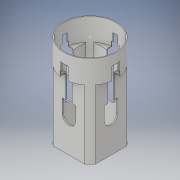
# Autodesk Inventor part: Hull2
Saved by Autodesk Inventor 2018.2 (Build 222227000, 227)
## iProperties
Created: 2017-12-27
Part Number: Hull2
Material: Generic
Document SubType Name: Modeling
Designer: Suchanek
Density: 1 g/cm^3
Appearance: Default
Mass: 15.1041 g
Surface Area: 312.787 cm^2
Volume: 15.1041 cm^3
Author: Suchanek
Autodesk Inventor part; units mm, degrees
ref_plane "YZ Plane" through (0, 0, 0) normal (1, 0, 0) x (0, 1, 0)
ref_plane "XZ Plane" through (0, 0, 0) normal (0, 1, 0) x (-1, 0, 0)
ref_plane "XY Plane" through (0, 0, 0) normal (0, 0, 1) x (1, 0, 0)
sketch "Sketch1" plane through (0, 0, 0) normal (0, 0, 1) x (1, 0, 0)
  line L0 (0, 0) -> (33, 0)
  line L1 (33, 0) -> (33, 1)
  line L2 (33, 1) -> (0, 1)
  line L3 (0, 1) -> (0, 0)
  line L4 (33, 0) -> (32, 0)
  line L5 (32, 0) -> (32, 115)
  line L6 (32, 115) -> (33, 115)
  line L7 (33, 115) -> (33, 0)
  line L8 (33, 115) -> (0, 115)
  line L9 (0, 115) -> (0, 115)
  line L10 (0, 115) -> (33, 115)
  line L11 (33, 115) -> (33, 115)
  line L12 (0, 115) -> (0, 1)
  line L13 (-5, 105) -> (5, 105)
  line L14 (5, 105) -> (5, 5)
  line L15 (5, 5) -> (-5, 5)
  line L16 (-5, 5) -> (-5, 105)
  dimension "d0" = 33
  dimension "d1" = 1
  dimension "d2" = 1
  dimension "d3" = 115
  dimension "d4" = 33
  dimension "d5" = 0
  dimension "d6" = 10
  dimension "d7" = 100
  dimension "d8" = 4
  constraints: 34 end point, 8 equal length, 4 perpendicular, 3 horizontal, 1 other
  measures "d0" distance of L2.end L1.end
  measures "d1" distance of L1.end L0.end
  measures "d2" distance of L5.end L6.end
  measures "d3" distance of L4.end L5.end
  measures "d4" distance of L10.end L9.end
  measures "d5" distance of L9.end L8.end
  measures "d6" distance of L14.end L15.end
  measures "d7" distance of L15.end L13.start
  measures "d8" distance from line of L1.end L15
sketch "Sketch2" plane through (0, 0, 0) normal (1, 0, 0) x (0, 1, 0)
  line L0 (102.5, 5) -> (5, 5)
  line L1 (5, 5) -> (5, -5)
  line L2 (5, -5) -> (102.5, -5)
  line L3 (102.5, -5) -> (102.5, 5)
  line L4 (0, 0) -> (0, -10)
  line L5 (0, 0) -> (115, 0)
  dimension "d9" = 10
  dimension "d10" = 5
  dimension "d12" = 115
  dimension "d13" = 10
  dimension "d14" = 97.5
  constraints: 12 end point, 2 horizontal, 2 parallel, 1 perpendicular, 1 vertical, 1 other
  measures "d9" distance of L4.start L4.end
  measures "d10" distance between parallel lines of L1 L4
  measures "d12" distance of L4.start L5.end
  measures "d13" distance between parallel lines of L0 L2
  measures "d14" distance of L1.end L2.end
extrude "Extrusion1" add sketch "Sketch2" along normal mid plane 10
revolve "Revolution1" add sketch "Sketch1" angle 360 about axis through (0, 115, 0) along (0, -1, 0) contours L3 L2 L5 L0 | L5 L2 L1 L0 | L5 L6 L7 L2
sketch "Sketch3" plane through (-5, 5, 5) normal (0, 0, 1) x (1, 0, 0)
  line L0 (0, 97.5) -> (10, 97.5) projected
  line L1 (10, 97.5) -> (10, 0) projected
  line L2 (0, 97.5) -> (10, 97.5)
  line L3 (10, 97.5) -> (10, 0)
  line L4 (10, 0) -> (0, 0)
  line L5 (0, 0) -> (0, 97.5)
  point P0 (5, -5)
  dimension "d18" = 97.5
  constraints: 8 end point, 2 parallel, 1 horizontal, 1 perpendicular
  measures "d18" distance of L2.end L1.end
extrude "Extrusion2" cut sketch "Sketch3" along normal mid plane 200
sketch "Sketch4" plane through (5, 0, 0) normal (1, 0, 0) x (0, 0, -1)
  line L0 (-5, 102.5) -> (-5, 5) projected
  line L1 (-5, 102.5) -> (5, 102.5)
  line L2 (5, 102.5) -> (5, 5)
  line L3 (5, 5) -> (-5, 5)
  line L4 (-5, 5) -> (-5, 102.5)
  point P0 (0, 0)
  dimension "d21" = 10
  dimension "d70" = 97.5
  constraints: 8 end point, 2 parallel, 1 horizontal, 1 perpendicular, 1 point on line
  measures "d21" distance of L2.end L3.end
  measures "d70" distance between parallel lines of L3 L1
extrude "Extrusion3" cut sketch "Sketch4" along normal mid plane 200
sketch "Sketch5" plane through (-32.619013, 5, -5) normal (0, 0, 1) x (1, 0, 0)
  line L0 (65.238026, 97.5) -> (64.225974, 97.5)
  line L1 (65.238026, 97.5) -> (55.238026, 97.5)
  line L2 (55.238026, 97.5) -> (55.238026, 87.5)
  line L3 (55.238026, 87.5) -> (65.238026, 87.5)
  line L4 (65.238026, 87.5) -> (65.238026, 97.5)
  line L5 (0, 97.5) -> (-0.380987, 97.5)
  line L6 (0, 97.5) -> (10, 97.5)
  line L7 (10, 97.5) -> (10, 87.5)
  line L8 (10, 87.5) -> (0, 87.5)
  line L9 (0, 87.5) -> (0, 97.5)
  circle A0 centre (7.5, 90) radius 1
  circle A1 centre (57.738026, 90) radius 1
  point P0 (32.619013, -5)
  dimension "d26" = 10
  dimension "d27" = 10
  dimension "d56" = 10
  dimension "d57" = 10
  dimension "d58" = 2
  dimension "d59" = 2.5
  dimension "d60" = 2.5
  dimension "d61" = 2
  dimension "d62" = 2.5
  dimension "d63" = 2.5
  constraints: 16 end point, 4 parallel, 2 centre point, 2 horizontal, 2 perpendicular
  measures "d26" distance of L3.end L2.end
  measures "d27" distance of L2.end L1.end
  measures "d56" distance of L7.end L8.end
  measures "d57" distance of L6.end L7.end
  measures "d58" diameter of A0
  measures "d59" distance from line of L7 A0.centre
  measures "d60" distance from line of L8 A0.centre
  measures "d61" diameter of A1
  measures "d62" distance from line of A1.centre L2
  measures "d63" distance from line of A1.centre L3
extrude "Extrusion4" add sketch "Sketch5" along normal blind 2
sketch "Sketch7" plane through (0, 1, 0) normal (0, 1, 0) x (1, 0, 0)
  line L0 (0, 0) -> (-26.5, 0)
  line L1 (-26.5, 0) -> (-26.5, 26.5)
  line L2 (-26.5, 26.5) -> (0, 26.5)
  line L3 (0, 26.5) -> (0, 0)
  line L4 (-26.5, 26.5) -> (26.5, 26.5)
  line L5 (26.5, 26.5) -> (26.5, 33.5)
  line L6 (26.5, 33.5) -> (-26.5, 33.5)
  line L7 (-26.5, 33.5) -> (-26.5, 26.5)
  line L8 (26.5, 26.5) -> (33.5, 26.5)
  line L9 (33.5, 26.5) -> (33.5, -26.5)
  line L10 (33.5, -26.5) -> (26.5, -26.5)
  line L11 (26.5, -26.5) -> (26.5, 26.5)
  line L12 (-26.5, 26.5) -> (-33.5, 26.5)
  line L13 (-33.5, 26.5) -> (-33.5, -26.5)
  line L14 (-33.5, -26.5) -> (-26.5, -26.5)
  line L15 (-26.5, -26.5) -> (-26.5, 26.5)
  line L16 (-26.5, -26.5) -> (26.5, -26.5)
  line L17 (26.5, -26.5) -> (26.5, -33.5)
  line L18 (26.5, -33.5) -> (-26.5, -33.5)
  line L19 (-26.5, -33.5) -> (-26.5, -26.5)
  dimension "d36" = 26.5
  dimension "d37" = 26.5
  dimension "d38" = 53
  dimension "d39" = 7
  dimension "d40" = 7
  dimension "d41" = 53
  dimension "d42" = 7
  dimension "d43" = 53
  dimension "d44" = 53
  dimension "d45" = 7
  constraints: 40 end point, 10 parallel, 5 horizontal, 5 perpendicular
  measures "d36" distance of L1.end L2.end
  measures "d37" distance of L0.end L1.end
  measures "d38" distance of L6.end L5.end
  measures "d39" distance of L5.end L4.end
  measures "d40" distance of L9.end L10.end
  measures "d41" distance of L8.end L9.end
  measures "d42" distance of L14.end L13.end
  measures "d43" distance of L13.end L12.end
  measures "d44" distance of L17.end L18.end
  measures "d45" distance of L16.end L17.end
extrude "Extrusion6" cut sketch "Sketch7" along normal blind 85 and the other way blind 5 contours L15 L14 L13 L12 L1 | L2 L7 L6 L5 L4 | L16 L17 L18 L19 | L8 L9 L10 L11
sketch "Sketch8" plane through (-17.937391, 1, 26.5) normal (0, 1, 0) x (1, 0, 0)
  point P0 (17.937391, 26.5)
sketch "Sketch9" plane through (-17.937391, 1, 26.5) normal (0, 1, 0) x (1, 0, 0)
  line L0 (1.437391, 43) -> (34.437391, 43)
  line L1 (34.437391, 43) -> (34.437391, 10)
  line L2 (34.437391, 10) -> (1.437391, 10)
  line L3 (1.437391, 10) -> (1.437391, 43)
  line L4 (35.874782, 53) -> (0, 53)
  line L5 (-8.562609, 6.83404) -> (-8.562609, 46.16596)
  line L6 (0, 0) -> (35.874782, 0)
  line L7 (44.437391, 8.562609) -> (44.437391, 44.437391)
  point P0 (17.937391, 26.5)
  dimension "d50" = 10
  dimension "d51" = 10
  dimension "d52" = 10
  dimension "d53" = 10
  constraints: 8 end point, 2 parallel, 1 horizontal, 1 perpendicular
  measures "d50" distance between parallel lines of L4 L0
  measures "d51" distance between parallel lines of L5 L3
  measures "d52" distance between parallel lines of L6 L2
  measures "d53" distance between parallel lines of L7 L1
extrude "Extrusion7" cut sketch "Sketch9" against normal blind 10
pattern_circular "Circular Pattern1" count 4 over 360 about axis through (0, 57.5, 0) along (0, -1, 0) of "Extrusion4"
sketch "Náčrt13" plane through (0, 115, 0) normal (0, 1, 0) x (1, 0, 0)
  point P0 (0, 0)
sketch "Náčrt14" plane through (-19.66596, 0, -26.5) normal (0, -1, 0) x (1, 0, 0)
  line L0 (-6.83404, 8.562609) -> (-6.83404, 44.437391)
  line L1 (-5.33404, 26.5) -> (-5.33404, 47.151249)
  arc A0 (-6.83404, 44.437391) -> (-6.83404, 8.562609) centre (19.66596, 26.5) ccw
  line L2 (-5.33404, 47.151249) -> (-6.83404, 44.437391)
  arc A1 (-11.941001, 21.5) -> (-6.83404, 8.562609) centre (19.66596, 26.5) ccw
  line L3 (-6.83404, 44.437391) -> (-6.83404, 8.562609)
  line L4 (-6.83404, 8.562609) -> (-5.33404, 4.959341)
  circle A2 centre (19.66596, 26.5) radius 33
  line L5 (-5.33404, 4.959341) -> (-5.33404, 26.5)
  point P0 (-11.042345, 35.5)
  point P1 (-11.042345, 17.5)
  dimension "d88" = 25
  constraints: 10 end point, 2 parallel, 1 point on line, 1 vertical, 2 other
  measures "d88" distance of point (19.666, 26.5) L1.start
extrude "Vysunutí9" add sketch "Náčrt14" against normal blind 87 contours L0 L2 L1 L5 L4
sketch "Náčrt15" plane through (0, 86, 0) normal (0, -1, 0) x (1, 0, 0)
  point P0 (0, 0)
sketch "Náčrt16" plane through (0, 86, 0) normal (0, -1, 0) x (1, 0, 0)
  line L0 (-31.606961, 5) -> (-32.619013, 5)
  arc A0 (-26.5, 19.66596) -> (-32.619013, 5) centre (0, 0) ccw
  line L1 (-26.5, 5) -> (-32.619013, 5)
  line L2 (-32.619013, 5) -> (-26.5, 5)
  line L3 (-26.5, 19.66596) -> (-26.5, 17.937391)
  line L4 (-26.5, 19.66596) -> (-32.619013, 5)
  line L5 (-26.5, 5) -> (-26.5, 19.66596)
  point P0 (0, 0)
  constraints: 8 end point, 1 collinear, 1 perpendicular, 1 point on line
extrude "Vysunutí10" add sketch "Náčrt16" against normal blind 1 contours L0 L4 L3 L5 L1
sketch "Náčrt17" plane through (0, 86, 0) normal (0, -1, 0) x (1, 0, 0)
  line L0 (-26.5, -17.937391) -> (-26.5, -19.66596)
  line L1 (-26.5, -5) -> (-26.5, -19.66596)
  line L2 (-26.5, -19.66596) -> (-30.211599, -12.140082)
  line L3 (-30.211599, -12.140082) -> (-31.970794, -5)
  line L4 (-31.970794, -5) -> (-26.5, -5)
  point P0 (0, 0)
  constraints: 8 end point, 1 perpendicular, 1 vertical
extrude "Vysunutí11" add sketch "Náčrt17" against normal blind 1
sketch "Náčrt18" plane through (-19.66596, 0, -26.5) normal (0, -1, 0) x (1, 0, 0)
  line L0 (0, 1.5) -> (41.20662, 1.5)
  circle A0 centre (19.66596, 26.5) radius 33
  line L1 (37.603352, 0) -> (1.728569, 0)
  line L2 (41.20662, 1.5) -> (37.603352, 0)
  line L3 (37.603352, 0) -> (1.728569, 0)
  line L4 (0, 1.5) -> (-1.874699, 1.5)
  line L5 (0, 0) -> (1.728569, 0)
  line L6 (-1.874699, 1.5) -> (1.728569, 0)
  dimension "d95" = 1.5
  constraints: 10 end point, 2 horizontal, 2 point on circle, 1 collinear
  measures "d95" distance of L5.start L0.start
extrude "Vysunutí12" add sketch "Náčrt18" against normal blind 87 contours L0 L2 L1 L6 L4
sketch "Náčrt19" plane through (0, 86, 0) normal (0, -1, 0) x (1, 0, 0)
  line L0 (-19.66596, -26.5) -> (-17.937391, -26.5)
  line L1 (-5, -26.5) -> (-19.66596, -26.5)
  line L2 (-19.66596, -26.5) -> (-9.21923, -31.085485)
  line L3 (-9.21923, -31.085485) -> (-5.463084, -31.92763)
  line L4 (-5.463084, -31.92763) -> (-5, -32.031455)
  line L5 (-5, -32.031455) -> (-5, -26.5)
  line L6 (17.937391, -26.5) -> (19.66596, -26.5)
  line L7 (18.386912, -26.5) -> (11.546452, -30.567242)
  line L8 (11.546452, -30.567242) -> (5, -32.031455)
  line L9 (5, -31.606961) -> (5, -26.5)
  line L10 (5, -32.031455) -> (5, -26.5)
  line L11 (5, -26.5) -> (18.386912, -26.5)
  point P0 (0, 0)
  constraints: 18 end point, 3 point on line, 2 collinear, 1 perpendicular, 1 vertical
extrude "Vysunutí13" add sketch "Náčrt19" against normal blind 1
sketch "Náčrt23" plane through (-19.66596, 0, 26.5) normal (0, -1, 0) x (1, 0, 0)
  line L0 (1.728569, 0) -> (0, 0)
  line L1 (-1.645269, -1.5) -> (1.728569, 0)
  line L2 (-1.645269, -1.5) -> (40.94385, -1.5)
  line L3 (40.94385, -1.5) -> (37.766415, 0)
  line L4 (39.331921, 0) -> (0, 0)
  line L5 (1.728569, 0) -> (37.766415, 0)
  line L6 (37.766415, 0) -> (1.728569, 0)
  line L7 (46.16596, -8.562609) -> (46.16596, -6.83404)
  line L8 (44.66596, -5.41272) -> (46.16596, -8.562609)
  line L9 (46.16596, -8.562609) -> (46.16596, -44.95022)
  line L10 (46.16596, -46.16596) -> (46.16596, -6.83404)
  line L11 (44.66596, -5.41272) -> (44.66596, -46.868472)
  line L12 (44.66596, -46.868472) -> (46.16596, -44.95022)
  point P0 (19.66596, -26.5)
  constraints: 18 end point, 2 collinear, 2 point on line, 1 horizontal, 1 vertical
extrude "Vysunutí14" add sketch "Náčrt23" against normal blind 87
sketch "Náčrt24" plane through (0, 86, 0) normal (0, -1, 0) x (1, 0, 0)
  line L0 (26.5, -19.66596) -> (26.5, -17.937391)
  line L1 (26.5, -5) -> (26.5, -18.550009)
  line L2 (26.5, -18.550009) -> (29.448278, -13.727211)
  line L3 (29.448278, -13.727211) -> (31.961082, -6.366097)
  line L4 (31.961082, -6.366097) -> (31.961082, -5)
  line L5 (31.961082, -5) -> (26.5, -5)
  line L6 (26.5, -5) -> (26.5, -18.550009)
  line L7 (26.5, -19.66596) -> (26.5, -17.937391)
  line L8 (26.5, 17.937391) -> (26.5, 19.66596)
  line L9 (26.5, 5) -> (26.5, 19.66596)
  line L10 (26.5, 19.66596) -> (30.063658, 11.946034)
  line L11 (30.063658, 11.946034) -> (31.704673, 7.086974)
  line L12 (31.704673, 7.086974) -> (32.613643, 5)
  line L13 (32.613643, 5) -> (26.5, 5)
  line L14 (5, 31.606961) -> (5, 32.619013)
  line L15 (-17.937391, 26.5) -> (17.937391, 26.5)
  line L16 (5, 26.5) -> (17.937391, 26.5)
  line L17 (17.937391, 26.5) -> (15.646086, 28.489705)
  line L18 (15.646086, 28.489705) -> (11.215549, 30.544064)
  line L19 (11.215549, 30.544064) -> (7.103364, 31.916843)
  line L20 (7.103364, 31.916843) -> (5, 32.619013)
  line L21 (5, 32.619013) -> (5, 26.5)
  line L22 (5, 32.619013) -> (5, 26.5)
  arc A0 (17.937391, 26.5) -> (31.606961, -5) centre (0, 0) ccw
  line L23 (17.937391, 26.5) -> (5, 26.5)
  line L24 (-13.573908, 29.516885) -> (-18.801676, 26.5)
  line L25 (-17.937391, 26.5) -> (-19.66596, 26.5)
  line L26 (-5, 32.619013) -> (-5, 31.606961)
  line L27 (-5, 26.5) -> (-18.801676, 26.5)
  line L28 (-13.573908, 29.516885) -> (-5, 32.177274)
  line L29 (-5, 32.105954) -> (-5, 26.5)
  point P0 (0, 0)
  point P1 (26.5, -9)
  point P2 (26.5, 9)
  point P3 (9, 26.5)
  point P4 (9, 30.708305)
  constraints: 46 end point, 4 perpendicular, 3 horizontal, 2 collinear, 2 point on line, 2 vertical, 1 midpoint, 1 parallel
extrude "Vysunutí15" add sketch "Náčrt24" against normal blind 1 contours L0 A0 L5 L4 L3 L2 | L1 L5 A0 | L8 L10 L11 L12 L13 L9 | A0 L15 L21 | L14 L20 L19 L18 L17 A0 | L29 L15 A0 | A0 L25 L24 L28 L26
sketch "Náčrt25" plane through (-19.66596, 0, 26.5) normal (0, 0, 1) x (1, 0, 0)
  line L0 (3.16596, 1) -> (36.16596, 1)
  line L1 (19.66596, 1) -> (24.16596, 1)
  line L2 (24.16596, 1) -> (15.16596, 1)
  line L3 (14.66596, 87) -> (24.66596, 87)
  line L4 (15.16596, 87) -> (24.16596, 87)
  line L5 (19.66596, 87) -> (23.66596, 87)
  line L6 (23.66596, 87) -> (15.66596, 87)
  line L7 (19.66596, 1) -> (19.66596, 41)
  circle A0 centre (19.66596, 41) radius 8.5
  line L8 (11.16596, 41) -> (11.16596, 58)
  line L9 (11.16596, 58) -> (28.16596, 58)
  line L10 (28.16596, 58) -> (28.16596, 41)
  line L11 (15.66596, 87) -> (15.66596, 58)
  line L12 (23.66596, 87) -> (23.66596, 58)
  point P0 (19.66596, 0)
  dimension "d114" = 4
  dimension "d115" = 8
  dimension "d116" = 40
  dimension "d117" = 17
  dimension "d118" = 17
  constraints: 22 end point, 7 point on line, 5 perpendicular, 2 midpoint, 2 point on circle, 1 centre point, 1 coincident, 1 tangent, 1 vertical
  measures "d114" distance of L5.start L5.end
  measures "d115" distance of L5.end L6.end
  measures "d116" distance of L1.start L7.end
  measures "d117" diameter of A0
  measures "d118" distance of L8.start L8.end
extrude "Vysunutí16" cut sketch "Náčrt25" against normal blind 160
sketch "Náčrt26" plane through (26.5, 0, 19.66596) normal (1, 0, 0) x (0, 0, -1)
  line L0 (44.66596, 87) -> (46.16596, 87)
  line L1 (19.66596, 87) -> (23.66596, 87)
  line L2 (23.66596, 87) -> (15.66596, 87)
  line L3 (-0.309024, 1) -> (39.640945, 1)
  line L4 (19.66596, 1) -> (19.66596, 41)
  circle A0 centre (19.66596, 41) radius 8.5
  line L5 (11.16596, 41) -> (11.16596, 58)
  line L6 (28.16596, 41) -> (28.16596, 58)
  line L7 (28.16596, 58) -> (11.16596, 58)
  line L8 (15.66596, 87) -> (15.66596, 58)
  line L9 (23.66596, 87) -> (23.66596, 58)
  point P0 (19.66596, 0)
  point P1 (4.66596, 87)
  point P2 (34.66596, 87)
  dimension "d121" = 4
  dimension "d122" = 8
  dimension "d123" = 40
  dimension "d124" = 17
  dimension "d125" = 17
  constraints: 16 end point, 5 point on line, 3 perpendicular, 3 vertical, 2 point on circle, 1 centre point, 1 coincident, 1 midpoint
  measures "d121" distance of L1.start L1.end
  measures "d122" distance of L1.end L2.end
  measures "d123" distance of L4.start L4.end
  measures "d124" diameter of A0
  measures "d125" distance of L5.start L5.end
extrude "Vysunutí17" cut sketch "Náčrt26" against normal blind 160
sketch "Náčrt28" plane through (0, 115, 0) normal (0, 1, 0) x (1, 0, 0)
  circle A0 centre (0, 0) radius 32
  constraints: 1 centre point, 1 coincident
extrude "Vysunutí18" cut sketch "Náčrt28" against normal blind 28
body "Solid1"
